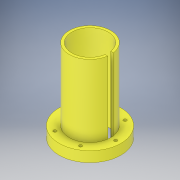
# Autodesk Inventor part: ExternalStationaryOuterRingOld
Saved by Autodesk Inventor 2019.3 (Build 233278000, 278)
## iProperties
Created: 2018-12-30
Part Number: ExternalStationaryOuterRingOld
Material: LCP Plastic
Document SubType Name: Modeling
Designer: steele
Density: 1.626 g/cm^3
Appearance: Smooth - Yellow
Author: steele
Autodesk Inventor part; units mm, degrees
ref_plane "YZ Plane" through (0, 0, 0) normal (1, 0, 0) x (0, 1, 0)
ref_plane "XZ Plane" through (0, 0, 0) normal (0, 1, 0) x (-1, 0, 0)
ref_plane "XY Plane" through (0, 0, 0) normal (0, 0, 1) x (1, 0, 0)
sketch "Sketch1" plane through (0, 0, 0) normal (0, 1, 0) x (-1, 0, 0)
  circle A0 centre (0, 0) radius 22.479
  circle A1 centre (0, 0) radius 25.654
  dimension "d0" = 44.958
  dimension "d1" = 51.308
  constraints: 2 centre point, 2 coincident
  measures "d0" diameter of A0
  measures "d1" diameter of A1
extrude "Extrusion1" add sketch "Sketch1" against normal blind 101.6
sketch "Sketch7" plane through (0, -101.6, 0) normal (0, -1, 0) x (1, 0, 0)
  line L0 (0, 0) -> (25.654, 0) construction
  circle A0 centre (0, 0) radius 25.654 construction
  line L1 (19.304, 3.429) -> (19.304, -3.429)
  line L2 (19.304, -3.429) -> (25.654, -3.429)
  line L3 (25.654, -3.429) -> (25.654, 3.429)
  line L4 (25.654, 3.429) -> (19.304, 3.429)
  circle A1 centre (0, 0) radius 22.479 projected
  line L5 (19.304, 3.429) -> (25.654, -3.429) construction
  line L6 (19.304, -3.429) -> (25.654, 3.429) construction
  point P0 (20.2202, 0)
  point P1 (22.479, 0)
  dimension "d10" = 6.858
  dimension "d11" = 6.35
  constraints: 14 end point, 2 horizontal alignment, 2 midpoint, 2 parallel, 2 perpendicular, 1 horizontal, 1 point on line, 2 other
  measures "d10" distance of L2.end L3.end
  measures "d11" distance of L3.end L1.start
extrude "Extrusion2" cut sketch "Sketch7" against normal blind 101.6 contours L4 A1 L2 L1 | L4 L3 L2 A1 picked at (20.3623, 0)
sketch "Sketch8" plane through (0, -101.6, 0) normal (0, -1, 0) x (1, 0, 0)
  circle A0 centre (0, 0) radius 25.654
  circle A1 centre (0, 0) radius 38.1
  dimension "d14" = 51.308
  dimension "d15" = 76.2
  constraints: 2 centre point, 2 coincident
  measures "d14" diameter of A0
  measures "d15" diameter of A1
extrude "Extrusion3" add sketch "Sketch8" against normal blind 12.7
sketch "Sketch10" plane through (0, -101.6, 0) normal (0, -1, 0) x (1, 0, 0)
  circle A0 centre (31.75, 0) radius 2.4257
  circle A1 centre (15.875, 27.4963) radius 2.4257
  circle A2 centre (-15.875, 27.4963) radius 2.4257
  circle A3 centre (-31.75, 0) radius 2.4257
  circle A4 centre (-15.875, -27.4963) radius 2.4257
  circle A5 centre (15.875, -27.4963) radius 2.4257
  point P0 (0, 0)
  dimension "d30" = 4.8514
  dimension "d33" = 360
  constraints: 6 centre point, 13 other
  measures "d30" diameter of A0
extrude "Extrusion4" cut sketch "Sketch10" against normal blind 7.1374
sketch "Sketch11" plane through (31.75, -94.4626, 0) normal (0, -1, 0) x (1, 0, 0)
  point P0 (-31.75, 0)
  point P1 (0, 0)
  point P2 (-15.875, 27.4963)
  point P3 (-47.625, 27.4963)
  point P4 (-63.5, 0)
  point P5 (-47.625, -27.4963)
  point P6 (-15.875, -27.4963)
  dimension "d39" = 360
  constraints: 7 other
hole "Hole2" at (31.75, -94.4626, 0) at (15.875, -94.4626, 27.4963) at (-15.875, -94.4626, 27.4963) at (-31.75, -94.4626, 0) at (-15.875, -94.4626, -27.4963) at (15.875, -94.4626, -27.4963) direction (0, 1, 0) diameter 3.81 end through all clearance for "Flat Head Machine Screw (82)" size "#6" standard "Ansi Unified Screw Threads"
body "Solid1"
